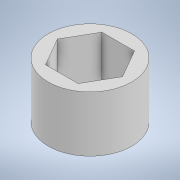
# Autodesk Inventor part: SP-003
Saved by Autodesk Inventor 2022.3 (Build 263350000, 350)
## iProperties
Created: 2023-01-29
Part Number: SP-003
Material: Generic
Document SubType Name: Modeling
Designer: 23kaltomare
Density: 1 g/cm^3
Appearance: Default
Author: 23kaltomare
Autodesk Inventor part; units mm, degrees
ref_plane "YZ Plane" through (0, 0, 0) normal (1, 0, 0) x (0, 1, 0)
ref_plane "XZ Plane" through (0, 0, 0) normal (0, 1, 0) x (-1, 0, 0)
ref_plane "XY Plane" through (0, 0, 0) normal (0, 0, 1) x (1, 0, 0)
sketch "Sketch1" plane through (0, 0, 0) normal (0, 1, 0) x (-1, 0, 0)
  line L0 (-3.7175, 6.4389) -> (3.7175, 6.4389)
  line L1 (3.7175, 6.4389) -> (7.435, 0)
  line L2 (7.435, 0) -> (3.7175, -6.4389)
  line L3 (3.7175, -6.4389) -> (-3.7175, -6.4389)
  line L4 (-3.7175, -6.4389) -> (-7.435, 0)
  line L5 (-7.435, 0) -> (-3.7175, 6.4389)
  circle A0 centre (0, 0) radius 9.525
  point P0 (5.5763, -3.2195)
  dimension "d0" = 12.8778
  dimension "d1" = 19.05
  constraints: 12 end point, 2 coincident, 1 centre point, 1 horizontal alignment, 1 midpoint, 13 other
  measures "d0" distance from line of point (5.576, -3.219) L5
  measures "d1" diameter of A0
extrude "Extrusion1" add sketch "Sketch1" along normal blind 12.7
body "Solid1"
